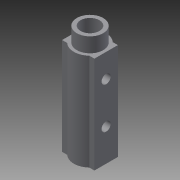
# Autodesk Inventor part: shaft_to_shaft_coupler
Saved by Autodesk Inventor 2015 (Build 190159000, 159)
## iProperties
Created: 2017-10-04
Part Number: shaft_to_shaft_coupler
Material: Generic
Document SubType Name: Modeling
Designer: Anshul
Density: 1 g/cm^3
Appearance: Default
Author: Anshul
Autodesk Inventor part; units mm, degrees
note: some values were not read from the file. Chosen so that the rebuilt part matches the saved one: sketch regions of "Extrusion3".
ref_plane "YZ Plane" through (0, 0, 0) normal (1, 0, 0) x (0, 1, 0)
ref_plane "XZ Plane" through (0, 0, 0) normal (0, 1, 0) x (-1, 0, 0)
ref_plane "XY Plane" through (0, 0, 0) normal (0, 0, 1) x (1, 0, 0)
sketch "Sketch1" plane through (0, 0, 0) normal (0, 1, 0) x (-1, 0, 0)
  circle A0 centre (0, 0) radius 3.2
  circle A1 centre (0, 0) radius 5.5
  line L0 (0, 0) -> (0, -3.2)
  line L1 (0, 0) -> (0, 4)
  line L2 (-3.7749, 4) -> (-5.5, 4)
  line L3 (-5.5, 4) -> (-5.5, -4)
  line L4 (-5.5, -4) -> (-3.7749, -4)
  line L5 (0, -4) -> (0, 0)
  line L6 (3.7749, -4) -> (5.5, -4)
  line L7 (5.5, -4) -> (5.5, 4)
  line L8 (5.5, 4) -> (3.7749, 4)
  circle A2 centre (0, 0) radius 4.5
  dimension "d0" = 6.4
  dimension "d1" = 11
  dimension "d13" = 4
  dimension "d14" = 8
  dimension "d15" = 8
  dimension "d18" = 9
  constraints: 18 end point, 4 coincident, 4 point on circle, 3 perpendicular, 3 point on line, 2 centre point, 2 vertical, 1 collinear, 1 vertical alignment, 2 other
  measures "d1" diameter of A1
  measures "d13" distance of L0.start L1.end
  measures "d14" distance of L2.end L3.end
  measures "d15" distance of L6.end L7.end
  measures "d18" diameter of A2
extrude "Extrusion3" add sketch "Sketch1" along normal blind 15 and the other way blind 18 contours A1 | L7 L6 A1 | A1 L8 L7 | A1 L3 L2 | L4 L3 A1 | A2
extrude "Extrusion4" add sketch "Sketch1" along normal blind 20 contours A2
sketch "Sketch3" plane through (5.5, -18, -4) normal (1, 0, 0) x (0, 0, -1)
  line L0 (0, 0) -> (0, 33) projected
  line L1 (0, 15) -> (-4, 15)
  line L2 (-4, 18) -> (-4, 11)
  line L3 (-4, 18) -> (-4, 25)
  circle A0 centre (-4, 25) radius 1.55
  circle A1 centre (-4, 11) radius 1.55
  dimension "d21" = 7
  dimension "d22" = 7
  dimension "d23" = 3.1
  dimension "d24" = 3.1
  constraints: 6 end point, 2 centre point, 2 coincident, 2 point on line, 1 horizontal, 1 perpendicular
  measures "d21" distance of L1.end L2.end
  measures "d22" distance of L1.end L3.end
  measures "d23" diameter of A0
  measures "d24" diameter of A1
extrude "Extrusion5" cut sketch "Sketch3" against normal blind 20
body "Solid2"
